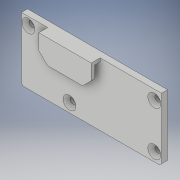
# Autodesk Inventor part: PowerMountingBracket
Saved by Autodesk Inventor 2019.3 (Build 233278000, 278)
## iProperties
Created: 2019-02-16
Part Number: PowerMountingBracket
Material: Generic
Document SubType Name: Modeling
Designer: mark
Density: 1 g/cm^3
Appearance: Default
Author: mark
Autodesk Inventor part; units mm, degrees
ref_plane "YZ Plane" through (0, 0, 0) normal (1, 0, 0) x (0, 1, 0)
ref_plane "XZ Plane" through (0, 0, 0) normal (0, 1, 0) x (-1, 0, 0)
ref_plane "XY Plane" through (0, 0, 0) normal (0, 0, 1) x (1, 0, 0)
sketch "Sketch1" plane through (0, 0, 0) normal (0, 0, 1) x (1, 0, 0)
  line L0 (0, 0) -> (80, 0)
  line L1 (80, 0) -> (80, 36)
  line L2 (80, 36) -> (0, 36)
  line L3 (0, 36) -> (0, 0)
  circle A0 centre (27.5, 30.464) radius 1.7
  circle A1 centre (27.5, 5.064) radius 1.7
  circle A2 centre (76, 30.464) radius 1.7
  circle A3 centre (76, 5.064) radius 1.7
  circle A4 centre (4, 31.365) radius 1.7
  circle A5 centre (19.558, 31.365) radius 1.7
  dimension "d0" = 36
  dimension "d1" = 80
  dimension "d2" = 3.4
  dimension "d3" = 3.4
  dimension "d4" = 3.4
  dimension "d5" = 3.4
  dimension "d6" = 3.4
  dimension "d7" = 3.4
  dimension "d8" = 5.536
  dimension "d10" = 5.536
  dimension "d11" = 48.5
  dimension "d12" = 25.4
  dimension "d13" = 48.5
  dimension "d14" = 25.4
  dimension "d16" = 15.558
  dimension "d17" = 4.635
  dimension "d18" = 4.635
  dimension "d39" = 4
  dimension "d40" = 4
  dimension "d41" = 4
  constraints: 8 end point, 6 centre point, 2 horizontal, 2 vertical
  measures "d0" distance between parallel lines of L0 L2
  measures "d1" distance between parallel lines of L1 L3
  measures "d2" diameter of A0
  measures "d3" diameter of A1
  measures "d4" diameter of A3
  measures "d5" diameter of A2
  measures "d6" diameter of A4
  measures "d7" diameter of A5
  measures "d8" distance from line of L2 A0.centre
  measures "d10" distance from line of L2 A2.centre
  measures "d11" distance of A0.centre A2.centre
  measures "d12" distance of A1.centre A0.centre
  measures "d13" distance of A1.centre A3.centre
  measures "d14" distance of A3.centre A2.centre
  measures "d16" distance of A5.centre A4.centre
  measures "d17" distance from line of L2 A4.centre
  measures "d18" distance from line of L2 A5.centre
  measures "d39" distance from line of A2.centre L1
  measures "d40" distance from line of A3.centre L1
  measures "d41" distance from line of A4.centre L3
extrude "Extrusion1" add sketch "Sketch1" along normal blind 3.5
sketch "Sketch2" plane through (0, 0, 3.5) normal (0, 0, 1) x (1, 0, 0)
  line L0 (15, 34) -> (45, 34)
  line L1 (45, 34) -> (45, 36)
  line L2 (45, 36) -> (15, 36)
  line L3 (15, 36) -> (15, 34)
  line L4 (80, 36) -> (0, 36) projected
  line L5 (0, 36) -> (0, 0) projected
  dimension "d22" = 2
  dimension "d23" = 15
  dimension "d24" = 30
  constraints: 8 end point, 1 collinear
  measures "d22" distance between parallel lines of L2 L0
  measures "d23" distance between parallel lines of L5 L3
  measures "d24" distance between parallel lines of L1 L3
extrude "Extrusion2" add sketch "Sketch2" along normal blind 5.1
sketch "Sketch3" plane through (15, 34, 3.5) normal (0, -1, 0) x (1, 0, 0)
  line L0 (0, 3.1) -> (30, 3.1)
  line L1 (30, 3.1) -> (30, 5.1)
  line L2 (30, 5.1) -> (0, 5.1)
  line L3 (0, 5.1) -> (0, 3.1)
  line L4 (0, 5.1) -> (30, 5.1) projected
  line L5 (0, 0) -> (0, 5.1) projected
  line L6 (30, 0) -> (30, 5.1) projected
  line L7 (-15, 0) -> (65, 0) projected
  point P0 (-15, -3.5)
  dimension "d27" = 3.1
  constraints: 8 end point, 3 collinear
  measures "d27" distance between parallel lines of L7 L0
extrude "Extrusion3" add sketch "Sketch3" along normal blind 11.75 contours L3 L2 L1 L0
chamfer "Chamfer1" distance 5 angle 45 2 edges at (15, 22.25, 7.6) (45, 22.25, 7.6)
chamfer "Chamfer2" distance 2 angle 45 6 edges at (25.8, 30.464, 3.5) (25.8, 5.064, 3.5) (74.3, 5.064, 3.5) (74.3, 30.464, 3.5) (2.3, 31.365, 3.5) (17.858, 31.365, 3.5)
chamfer "Chamfer3" distance 1 angle 45 2 edges at (0, 0, 1.75) (80, 0, 1.75)
body "Solid1"
